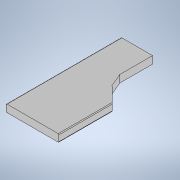
# Autodesk Inventor part: VerstaerkungHintenLinks
Saved by Autodesk Inventor 2020.3 (Build 243373010, 373A)
## iProperties
Created: 2021-02-13
Part Number: VerstaerkungHintenLinks
Material: Generisch
Document SubType Name: Modeling
Designer: Stefan
Density: 1 g/cm^3
Appearance: Vorgabe
Author: Stefan
Autodesk Inventor part; units mm, degrees
ref_plane "YZ Plane" through (0, 0, 0) normal (1, 0, 0) x (0, 1, 0)
ref_plane "XZ Plane" through (0, 0, 0) normal (0, 1, 0) x (-1, 0, 0)
ref_plane "XY Plane" through (0, 0, 0) normal (0, 0, 1) x (1, 0, 0)
sketch "Skizze1" plane through (0, 0, 0) normal (0, 1, 0) x (-1, 0, 0)
  line L0 (100.9437, 169.5604) -> (-41.0563, 169.5604)
  line L1 (-41.0563, 169.5604) -> (-41.0563, -140.4396)
  line L2 (-41.0563, -140.4396) -> (100.9437, -140.4396)
  line L3 (100.9437, -140.4396) -> (100.9437, 169.5604)
  point P0 (0, 0)
  dimension "d0" = 142
  dimension "d1" = 310
  constraints: 8 end point, 2 parallel, 1 horizontal, 1 perpendicular, 1 other
  measures "d0" distance of L1.end L2.end
  measures "d1" distance of L0.end L1.end
extrude "Extrusion1" add sketch "Skizze1" along normal blind 20
sketch "Skizze3" plane through (0, 20, 0) normal (0, 1, 0) x (1, 0, 0)
  line L0 (41.0563, -169.5604) -> (41.0563, 140.4396) projected
  line L1 (-100.9437, -169.5604) -> (41.0563, -169.5604) projected
  line L2 (41.0563, 140.4396) -> (-15.9437, 140.4396)
  line L3 (-15.9437, 140.4396) -> (-15.9437, -169.5604)
  line L4 (-15.9437, -169.5604) -> (41.0563, -169.5604)
  line L5 (41.0563, -169.5604) -> (41.0563, 140.4396)
  line L6 (-100.9437, 140.4396) -> (-100.9437, -169.5604) projected
  line L7 (-55.1017, 146.8416) -> (-0.3577, 14.6778)
  line L8 (0.4663, 14.6778) -> (101.62, -86.4759)
  line L9 (-0.3577, 14.6778) -> (0.4663, 14.6778)
  point P0 (0, 0)
  point P1 (-15.9437, 52.3058)
  point P2 (41.0563, -25.9122)
  dimension "d66" = 85
  dimension "d69" = 157.5
  dimension "d70" = 316.402
  dimension "d71" = 45.842
  dimension "d72" = 143.053
  dimension "d74" = 143.053
  dimension "d75" = 157.5
  dimension "d76" = 0
  dimension "d77" = 0.824
  constraints: 14 end point, 2 horizontal, 2 parallel, 2 point on line, 1 perpendicular
  measures "d66" distance between parallel lines of L6 L3
  measures "d69" angle of L0 L7
  measures "d70" distance from line of L1 L7.start
  measures "d71" distance from line of L6 L7.start
  measures "d72" distance of L7.start L7.end
  measures "d74" distance of L8.start L8.end
  measures "d75" angle of L7 L8
  measures "d76" vertical distance of L8.start L7.end
  measures "d77" distance of L8.start L7.end
extrude "Extrusion4" cut sketch "Skizze3" against normal through all contours L8 L9 L7 L3 L2 L0
fillet "Rundung1" radius 2 4 edges at (-100.9437, 20, 14.5604) (-100.9437, 0, 14.5604) (41.0563, 20, 97.7363) (41.0563, 0, 97.7363)
